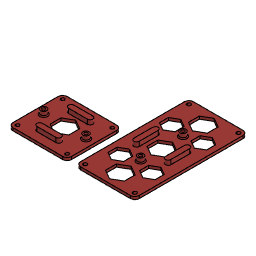
Lower Bay - SSR-40 DA (Autodesk Fusion 360 design; units mm, degrees)
Autodesk Fusion 360 part; units mm, degrees
derive "derive" from "Case Master - OmniBox v75"
sketch "Sketch1" plane through (0, 0, 0) normal (0, 0, 1) x (1, 0, 0)
  line L0 (-65, 70) -> (-10, 70) construction
  line L1 (-10, 70) -> (-10, 20) construction
  line L2 (-10, 20) -> (-65, 20) construction
  line L3 (-65, 20) -> (-65, 70) construction
  line L4 (-70, 20) -> (-70, 70)
  arc A0 (-65, 75) -> (-70, 70) centre (-65, 70) ccw
  arc A1 (-5, 70) -> (-10, 75) centre (-10, 70) ccw
  line L5 (-5, 70) -> (-5, 20)
  line L6 (-65, 75) -> (-10, 75)
  arc A2 (-70, 20) -> (-65, 15) centre (-65, 20) ccw
  line L7 (-10, 15) -> (-65, 15)
  arc A3 (-10, 15) -> (-5, 20) centre (-10, 20) ccw
  line L8 (-66.8, 70.25) -> (-66.8, 69.75)
  arc A4 (-66.8, 69.75) -> (-63.2, 69.75) centre (-65, 69.75) ccw
  line L9 (-63.2, 69.75) -> (-63.2, 70.25)
  arc A5 (-63.2, 70.25) -> (-66.8, 70.25) centre (-65, 70.25) ccw
  line L10 (-65, 70.25) -> (-65, 69.75) construction
  line L11 (-37.5, 75) -> (-37.5, 15) construction
  line L12 (-70, 45) -> (-5, 45) construction
  arc A6 (-66.8, 19.75) -> (-63.2, 19.75) centre (-65, 19.75) ccw
  line L13 (-66.8, 19.75) -> (-66.8, 20.25)
  arc A7 (-63.2, 20.25) -> (-66.8, 20.25) centre (-65, 20.25) ccw
  line L14 (-63.2, 20.25) -> (-63.2, 19.75)
  arc A8 (-8.2, 70.25) -> (-11.8, 70.25) centre (-10, 70.25) ccw
  line L15 (-8.2, 70.25) -> (-8.2, 69.75)
  arc A9 (-11.8, 69.75) -> (-8.2, 69.75) centre (-10, 69.75) ccw
  line L16 (-11.8, 69.75) -> (-11.8, 70.25)
  line L17 (-11.8, 20.25) -> (-11.8, 19.75)
  arc A10 (-8.2, 20.25) -> (-11.8, 20.25) centre (-10, 20.25) ccw
  line L18 (-8.2, 19.75) -> (-8.2, 20.25)
  arc A11 (-11.8, 19.75) -> (-8.2, 19.75) centre (-10, 19.75) ccw
  line L19 (70, 140) -> (70, 15) construction
  line L20 (70, 15) -> (5, 15) construction
  line L21 (5, 140) -> (70, 140) construction
  line L22 (5, 15) -> (5, 140) construction
  line L23 (10, 135) -> (65, 135) construction
  line L24 (65, 135) -> (65, 20) construction
  line L25 (65, 20) -> (10, 20) construction
  line L26 (10, 20) -> (10, 135) construction
  line L27 (65, 15) -> (10, 15)
  line L28 (5, 20) -> (5, 135)
  line L29 (10, 140) -> (65, 140)
  line L30 (70, 135) -> (70, 20)
  arc A12 (10, 140) -> (5, 135) centre (10, 135) ccw
  arc A13 (70, 135) -> (65, 140) centre (65, 135) ccw
  arc A14 (5, 20) -> (10, 15) centre (10, 20) ccw
  arc A15 (65, 15) -> (70, 20) centre (65, 20) ccw
  line L31 (8.1, 135.25) -> (8.1, 134.75)
  arc A16 (8.1, 134.75) -> (11.9, 134.75) centre (10, 134.75) ccw
  line L32 (11.9, 134.75) -> (11.9, 135.25)
  arc A17 (11.9, 135.25) -> (8.1, 135.25) centre (10, 135.25) ccw
  line L33 (10, 135.25) -> (10, 134.75) construction
  line L34 (37.5, 140) -> (37.5, 15) construction
  line L35 (5, 77.5) -> (70, 77.5) construction
  arc A18 (63.1, 134.75) -> (66.9, 134.75) centre (65, 134.75) ccw
  line L36 (63.1, 134.75) -> (63.1, 135.25)
  arc A19 (66.9, 135.25) -> (63.1, 135.25) centre (65, 135.25) ccw
  line L37 (66.9, 135.25) -> (66.9, 134.75)
  line L38 (66.9, 19.75) -> (66.9, 20.25)
  arc A20 (63.1, 19.75) -> (66.9, 19.75) centre (65, 19.75) ccw
  line L39 (63.1, 20.25) -> (63.1, 19.75)
  arc A21 (66.9, 20.25) -> (63.1, 20.25) centre (65, 20.25) ccw
  arc A22 (8.1, 19.75) -> (11.9, 19.75) centre (10, 19.75) ccw
  line L40 (8.1, 19.75) -> (8.1, 20.25)
  line L41 (11.9, 20.25) -> (11.9, 19.75)
  arc A23 (11.9, 20.25) -> (8.1, 20.25) centre (10, 20.25) ccw
  point P0 (-65, 70)
  point P1 (10, 135)
  point P2 (65, 135)
  point P3 (10, 20)
  point P4 (65, 20)
  point P5 (10, 135)
  dimension "d1" = 3.6
  dimension "d5" = 3.8
  constraint tangent L8 A4
  constraint tangent A4 L9
  constraint parallel L8 L9
  constraint tangent L9 A5
  constraint tangent L8 A5
  constraint vertical L10
  constraint coincident P0 L0.start
  constraint midpoint L10 P0
  constraint midpoint L6 L11.start
  constraint midpoint L7 L11.end
  constraint midpoint L4 L12.start
  constraint midpoint L5 L12.end
  constraint symmetric L8.start L12 A6.start
  constraint symmetric L8.end L12 L13.end
  constraint symmetric A4.end L12 A7.start
  constraint symmetric L9.end L12 A6.end
  constraint symmetric A4 L12 A7
  constraint symmetric A5 L12 A6
  constraint symmetric L8.start L11 A8.start
  constraint symmetric L8.end L11 L15.end
  constraint symmetric A4.end L11 A9.start
  constraint symmetric L9.end L11 A8.end
  constraint symmetric A4 L11 A9
  constraint symmetric A5 L11 A8
  constraint symmetric L11 A6.end L17.end
  constraint symmetric L11 A6.start L18.start
  constraint symmetric L11 A6 A11
  constraint symmetric L11 L13.end A10.start
  constraint symmetric L11 A7.start L17.start
  constraint symmetric L11 A7 A10
  constraint horizontal L23
  constraint vertical L24
  constraint horizontal L25
  constraint vertical L26
  constraint coincident P4 L24.end
  constraint coincident P5 P1
  constraint coincident L21 L29.start
  constraint parallel L25 L27
  constraint parallel L26 L28
  constraint parallel L23 L29
  constraint parallel L24 L30
  constraint coincident L21 L29.end
  constraint coincident P2 L23.end
  constraint coincident L22 L28.start
  constraint coincident P3 L25.end
  constraint tangent L31 A16
  constraint tangent A16 L32
  constraint parallel L31 L32
  constraint tangent L32 A17
  constraint tangent L31 A17
  constraint vertical L33
  constraint midpoint L33 P5
  constraint midpoint L21 L34.start
  constraint midpoint L20 L34.end
  constraint midpoint L28 L35.start
  constraint midpoint L19 L35.end
  constraint symmetric L31.start L34 A19.start
  constraint symmetric L31.end L34 A18.end
  constraint symmetric A16.end L34 A18.start
  constraint symmetric L32.end L34 L36.end
  constraint symmetric A16 L34 A18
  constraint symmetric A17 L34 A19
  constraint symmetric L31.start L35 A22.start
  constraint symmetric L31.end L35 L40.end
  constraint symmetric A16.end L35 L41.start
  constraint symmetric L32.end L35 A22.end
  constraint symmetric A16 L35 A23
  constraint symmetric A17 L35 A22
  constraint symmetric L35 A18.end L38.end
  constraint symmetric L35 A18.start L39.start
  constraint symmetric L35 A18 A21
  constraint symmetric L35 L36.end A20.start
  constraint symmetric L35 A19.start L38.start
  constraint symmetric L35 A19 A20
  measures "d1" diameter of A4
  measures "d5" diameter of A16
extrude "Extrude1" add sketch "Sketch1" along normal blind 3 contours L27 L28 L29 L30 A12 A13 A14 A15 makes body 1 in component "Long Tray"
extrude "Extrude1'" add sketch "Sketch1" along normal blind 3 separate body contours L4 A0 A1 L5 L6 A2 L7 A3 makes body 2 in component "Short Tray"
ref_plane "WorkPlane1" through (0, 0, 3) normal (0, 0, 1) x (1, 0, 0)
sketch "Sketch2" plane through (0, 0, 3) normal (0, 0, 1) x (-1, 0, 0)
  arc A0 (-66.9, -20.25) -> (-63.1, -20.25) centre (-65, -20.25) ccw
  line L0 (-66.9, -20.25) -> (-66.9, -19.75)
  arc A1 (-63.1, -19.75) -> (-66.9, -19.75) centre (-65, -19.75) ccw
  line L1 (-63.1, -19.75) -> (-63.1, -20.25)
  arc A2 (-11.9, -135.25) -> (-8.1, -135.25) centre (-10, -135.25) ccw
  line L2 (-11.9, -135.25) -> (-11.9, -134.75)
  arc A3 (-8.1, -134.75) -> (-11.9, -134.75) centre (-10, -134.75) ccw
  line L3 (-8.1, -134.75) -> (-8.1, -135.25)
  arc A4 (-8.1, -19.75) -> (-11.9, -19.75) centre (-10, -19.75) ccw
  line L4 (-8.1, -19.75) -> (-8.1, -20.25)
  arc A5 (-11.9, -20.25) -> (-8.1, -20.25) centre (-10, -20.25) ccw
  line L5 (-11.9, -20.25) -> (-11.9, -19.75)
  arc A6 (-63.1, -134.75) -> (-66.9, -134.75) centre (-65, -134.75) ccw
  line L6 (-63.1, -134.75) -> (-63.1, -135.25)
  arc A7 (-66.9, -135.25) -> (-63.1, -135.25) centre (-65, -135.25) ccw
  line L7 (-66.9, -135.25) -> (-66.9, -134.75)
  arc A8 (-5, -20) -> (-10, -15) centre (-10, -20) ccw
  line L8 (-10, -15) -> (-65, -15)
  arc A9 (-65, -15) -> (-70, -20) centre (-65, -20) ccw
  line L9 (-70, -20) -> (-70, -135)
  arc A10 (-70, -135) -> (-65, -140) centre (-65, -135) ccw
  line L10 (-65, -140) -> (-10, -140)
  arc A11 (-10, -140) -> (-5, -135) centre (-10, -135) ccw
  line L11 (-5, -135) -> (-5, -20)
  line L12 (-37.5, -140) -> (-37.5, -15) construction
  line L13 (-37.5, -77.5) -> (-37.5, -101) construction
  circle A12 centre (-37.5, -101) radius 1.8
  circle A13 centre (-37.5, -101) radius 3.4
  line L14 (-37.5, -77.5) -> (-15, -77.5) construction
  circle A14 centre (-37.5, -54) radius 3.4
  circle A15 centre (-37.5, -54) radius 1.8
  line L15 (-15, -77.5) -> (-20, -77.5) construction
  line L16 (-23, -67) -> (-23, -88)
  arc A16 (-23, -88) -> (-17, -88) centre (-20, -88) ccw
  line L17 (-17, -88) -> (-17, -67)
  arc A17 (-17, -67) -> (-23, -67) centre (-20, -67) ccw
  line L18 (-20, -67) -> (-20, -88) construction
  line L19 (-58, -88) -> (-58, -67)
  arc A18 (-52, -67) -> (-58, -67) centre (-55, -67) ccw
  line L20 (-52, -67) -> (-52, -88)
  arc A19 (-58, -88) -> (-52, -88) centre (-55, -88) ccw
  arc A20 (48, -30.5) -> (48, -24.5) centre (48, -27.5) ccw
  arc A21 (48, -65.5) -> (48, -59.5) centre (48, -62.5) ccw
  line L21 (37.5, -22.5) -> (37.5, -27.5) construction
  line L22 (48, -24.5) -> (27, -24.5)
  line L23 (48, -65.5) -> (27, -65.5)
  arc A22 (27, -59.5) -> (27, -65.5) centre (27, -62.5) ccw
  line L24 (37.5, -45) -> (61, -45) construction
  circle A23 centre (61, -45) radius 1.8
  circle A24 centre (14, -45) radius 3.4
  circle A25 centre (61, -45) radius 3.4
  arc A26 (27, -24.5) -> (27, -30.5) centre (27, -27.5) ccw
  line L25 (37.5, -45) -> (37.5, -22.5) construction
  circle A27 centre (14, -45) radius 1.8
  line L26 (27, -59.5) -> (48, -59.5)
  line L27 (27, -30.5) -> (48, -30.5)
  line L28 (27, -27.5) -> (48, -27.5) construction
  point P0 (-37.5, -77.5)
  point P1 (-20, -77.5)
  point P2 (37.5, -27.5)
  point P3 (37.5, -45)
  dimension "d17" = 23.5
  dimension "d18" = 3.6
  dimension "d19" = 1.6
  dimension "d20" = 5
  dimension "d39" = 23.5
  dimension "d40" = 3.6
  dimension "d41" = 5
  constraint midpoint L10 L12.start
  constraint midpoint L8 L12.end
  constraint midpoint L12 P0
  constraint coincident P0 L13.start
  constraint parallel L12 L13
  constraint coincident L13.end A12.centre
  constraint symmetric A12 L14 A15
  constraint symmetric A13 L14 A14
  constraint tangent L16 A16
  constraint tangent A16 L17
  constraint parallel L16 L17
  constraint tangent L17 A17
  constraint tangent L16 A17
  constraint perpendicular L14 L18
  constraint coincident P1 L15.end
  constraint midpoint L18 P1
  constraint symmetric L13 L16.start A18.start
  constraint symmetric L13 L16.end L20.end
  constraint symmetric L13 A16.end L19.start
  constraint symmetric L13 L17.end L19.end
  constraint symmetric L13 A16 A19
  constraint symmetric L13 A17 A18
  constraint coincident P3 L24.start
  constraint coincident L24.end A23.centre
  constraint symmetric A23 L25 A27
  constraint symmetric A24 A25 L25
  constraint tangent A20 L27
  constraint tangent A20 L22
  constraint parallel L22 L27
  constraint tangent L22 A26
  constraint tangent A26 L27
  constraint perpendicular L25 L28
  constraint coincident P2 L21.end
  constraint midpoint P2 L28
  constraint symmetric A22.start A26.end L24
  constraint symmetric A21.end A20.start L24
  constraint symmetric A21.start A20.end L24
  constraint symmetric L23.end L22.end L24
  constraint symmetric A20 A21 L24
  constraint symmetric A22 L24 A26
  constraint concentric A23 A25
  measures "d17" distance of P0 L13.end
  measures "d18" diameter of A12
  measures "d20" distance of L14.end P1
  measures "d39" distance of P3 L24.end
  measures "d40" diameter of A23
  measures "d41" distance of P2 L21.start
extrude "Extrude2" add sketch "Sketch2" along normal blind 5 contours A13 | A14 | L16 A16 L17 A17 | L19 A18 L20 A19 bodies 1 in component "Long Tray"
extrude "Extrude3" cut sketch "Sketch2" against normal blind 3 contours A12 | A15 | A23 | A27 bodies 1 in component "Long Tray"
sketch "Sketch3" plane through (0, 0, 3) normal (0, 0, 1) x (-1, 0, 0)
  circle A0 centre (-37.5, -101) radius 3.4
  line L0 (-17, -67) -> (-17, -88)
  arc A1 (-23, -88) -> (-17, -88) centre (-20, -88) ccw
  line L1 (-23, -88) -> (-23, -67)
  arc A2 (-17, -67) -> (-23, -67) centre (-20, -67) ccw
  arc A3 (-66.9, -20.25) -> (-63.1, -20.25) centre (-65, -20.25) ccw
  line L2 (-66.9, -20.25) -> (-66.9, -19.75)
  arc A4 (-63.1, -19.75) -> (-66.9, -19.75) centre (-65, -19.75) ccw
  line L3 (-63.1, -19.75) -> (-63.1, -20.25)
  arc A5 (-11.9, -135.25) -> (-8.1, -135.25) centre (-10, -135.25) ccw
  line L4 (-11.9, -135.25) -> (-11.9, -134.75)
  arc A6 (-8.1, -134.75) -> (-11.9, -134.75) centre (-10, -134.75) ccw
  line L5 (-8.1, -134.75) -> (-8.1, -135.25)
  arc A7 (-8.1, -19.75) -> (-11.9, -19.75) centre (-10, -19.75) ccw
  line L6 (-8.1, -19.75) -> (-8.1, -20.25)
  arc A8 (-11.9, -20.25) -> (-8.1, -20.25) centre (-10, -20.25) ccw
  line L7 (-11.9, -20.25) -> (-11.9, -19.75)
  arc A9 (-63.1, -134.75) -> (-66.9, -134.75) centre (-65, -134.75) ccw
  line L8 (-63.1, -134.75) -> (-63.1, -135.25)
  arc A10 (-66.9, -135.25) -> (-63.1, -135.25) centre (-65, -135.25) ccw
  line L9 (-66.9, -135.25) -> (-66.9, -134.75)
  arc A11 (-5, -20) -> (-10, -15) centre (-10, -20) ccw
  line L10 (-10, -15) -> (-65, -15)
  arc A12 (-65, -15) -> (-70, -20) centre (-65, -20) ccw
  line L11 (-70, -20) -> (-70, -135)
  arc A13 (-70, -135) -> (-65, -140) centre (-65, -135) ccw
  line L12 (-65, -140) -> (-10, -140)
  arc A14 (-10, -140) -> (-5, -135) centre (-10, -135) ccw
  line L13 (-5, -135) -> (-5, -20)
  line L14 (-52, -67) -> (-52, -88)
  arc A15 (-58, -88) -> (-52, -88) centre (-55, -88) ccw
  line L15 (-58, -88) -> (-58, -67)
  arc A16 (-52, -67) -> (-58, -67) centre (-55, -67) ccw
  circle A17 centre (-37.5, -54) radius 3.4
  line L16 (-37.5, -140) -> (-37.5, -15) construction
  line L17 (-37.5, -89.5) -> (-27.1077, -83.5)
  line L18 (-27.1077, -83.5) -> (-27.1077, -71.5)
  line L19 (-27.1077, -71.5) -> (-37.5, -65.5)
  line L20 (-37.5, -65.5) -> (-47.8923, -71.5)
  line L21 (-47.8923, -71.5) -> (-47.8923, -83.5)
  line L22 (-47.8923, -83.5) -> (-37.5, -89.5)
  line L23 (-37.5, -77.5) -> (-5, -77.5) construction
  line L24 (-47.8923, -129.5) -> (-37.5, -135.5)
  line L25 (-37.5, -135.5) -> (-27.1077, -129.5)
  line L26 (-27.1077, -129.5) -> (-27.1077, -117.5)
  line L27 (-27.1077, -117.5) -> (-37.5, -111.5)
  line L28 (-37.5, -111.5) -> (-47.8923, -117.5)
  line L29 (-47.8923, -117.5) -> (-47.8923, -129.5)
  line L30 (-47.8923, -37.5) -> (-37.5, -43.5)
  line L31 (-37.5, -43.5) -> (-27.1077, -37.5)
  line L32 (-27.1077, -37.5) -> (-27.1077, -25.5)
  line L33 (-27.1077, -25.5) -> (-37.5, -19.5)
  line L34 (-37.5, -19.5) -> (-47.8923, -25.5)
  line L35 (-47.8923, -25.5) -> (-47.8923, -37.5)
  line L36 (-20, -91) -> (-20, -106) construction
  line L37 (-20, -116) -> (-11.3397, -111)
  line L38 (-11.3397, -111) -> (-11.3397, -101)
  line L39 (-11.3397, -101) -> (-20, -96)
  line L40 (-20, -96) -> (-28.6603, -101)
  line L41 (-28.6603, -101) -> (-28.6603, -111)
  line L42 (-28.6603, -111) -> (-20, -116)
  line L43 (-63.6603, -111) -> (-63.6603, -101)
  line L44 (-63.6603, -101) -> (-55, -96)
  line L45 (-55, -96) -> (-46.3397, -101)
  line L46 (-46.3397, -101) -> (-46.3397, -111)
  line L47 (-46.3397, -111) -> (-55, -116)
  line L48 (-55, -116) -> (-63.6603, -111)
  line L49 (-63.6603, -44) -> (-63.6603, -54)
  line L50 (-63.6603, -54) -> (-55, -59)
  line L51 (-55, -59) -> (-46.3397, -54)
  line L52 (-46.3397, -54) -> (-46.3397, -44)
  line L53 (-46.3397, -44) -> (-55, -39)
  line L54 (-55, -39) -> (-63.6603, -44)
  line L55 (-11.3397, -44) -> (-11.3397, -54)
  line L56 (-11.3397, -54) -> (-20, -59)
  line L57 (-20, -59) -> (-28.6603, -54)
  line L58 (-28.6603, -54) -> (-28.6603, -44)
  line L59 (-20, -39) -> (-11.3397, -44)
  line L60 (-28.6603, -44) -> (-20, -39)
  line L61 (27.1077, -51) -> (37.5, -57)
  line L62 (37.5, -57) -> (47.8923, -51)
  line L63 (47.8923, -51) -> (47.8923, -39)
  line L64 (47.8923, -39) -> (37.5, -33)
  line L65 (37.5, -33) -> (27.1077, -39)
  line L66 (27.1077, -39) -> (27.1077, -51)
  point P0 (-37.5, -77.5)
  point P1 (-20, -106)
  dimension "d25" = 12
  dimension "d28" = 0
  dimension "d29" = 46
  dimension "d34" = 15
  dimension "d35" = 10
  constraint midpoint L12 L16.start
  constraint midpoint L10 L16.end
  constraint midpoint L16 P0
  constraint coincident L16 L17.start
  constraint coincident P0 L23.start
  constraint coincident L13 L23.end
  constraint horizontal L23
  constraint midpoint A1 L36.start
  constraint parallel L1 L36
  constraint coincident P1 L36.end
  constraint symmetric L16 L37.start L47.end
  constraint symmetric L16 L37.end L43.start
  constraint symmetric L16 L38.end L43.end
  constraint symmetric L16 L39.end L44.end
  constraint symmetric L16 L40.end L45.end
  constraint symmetric L16 L41.end L46.end
  constraint symmetric L23 L37.start L59.start
  constraint symmetric L23 L37.end L55.start
  constraint symmetric L23 L38.end L55.end
  constraint symmetric L23 L39.end L56.end
  constraint symmetric L23 L40.end L57.end
  constraint symmetric L23 L41.end L58.end
  constraint symmetric L23 L43.start L49.start
  constraint symmetric L23 L43.end L49.end
  constraint symmetric L23 L44.end L50.end
  constraint symmetric L23 L45.end L51.end
  constraint symmetric L23 L46.end L52.end
  constraint symmetric L23 L47.end L53.end
  measures "d25" distance of L17.start P0
  measures "d34" distance of L36.start P1
  measures "d35" distance of L37.start P1
extrude "Extrude4" cut sketch "Sketch3" against normal blind 3 contours L17 L18 L19 L20 L21 L22 | L24 L25 L26 L27 L28 L29 | L30 L31 L32 L33 L34 L35 | L37 L38 L39 L40 L41 L42 | L43 L44 L45 L46 L47 L48 | L49 L50 L51 L52 L53 L54 | L55 L56 L57 L58 L59 L60 bodies 1 in component "Long Tray"
extrude "Extrude2'" cut sketch "Sketch2" against normal blind 3 contours A23 | A27 bodies 2 in component "Short Tray"
extrude "Extrude3'" cut sketch "Sketch3" against normal blind 3 contours L61 L62 L63 L64 L65 L66 bodies 2 in component "Short Tray"
extrude "Extrude4'" add sketch "Sketch2" along normal blind 5 contours A20 L22 A26 L27 | A21 L23 A22 L26 | A24 | A25 bodies 2 in component "Short Tray"
fillet "Fillet1" radius 1 2 edges at (-12.7705, 48.1699, 3) (-59.7705, 48.1699, 3) on bodies 2 in component "Short Tray"
fillet "Fillet1'" radius 1 2 edges at (40.6699, 52.7705, 3) (40.6699, 99.7705, 3) on bodies 1 in component "Long Tray"
component "Long Tray" placed x (1, 0, 0) y (0, 1, 0) z (0, 0, 1) at (0, 0, 0)
component "Short Tray" placed x (1, 0, 0) y (0, 1, 0) z (0, 0, 1) at (0, 0, 0)
equation "large_m4 = 4.6 mm"
equation "small_m4 = 3.8 mm"
equation "large_m3 = 3.6 mm"
equation "small_m3 = 2.8 mm"
equation "d17 = ( 47 / 2 ) * 1 mm"
equation "d39 = ( 47 / 2 ) * 1 mm"
